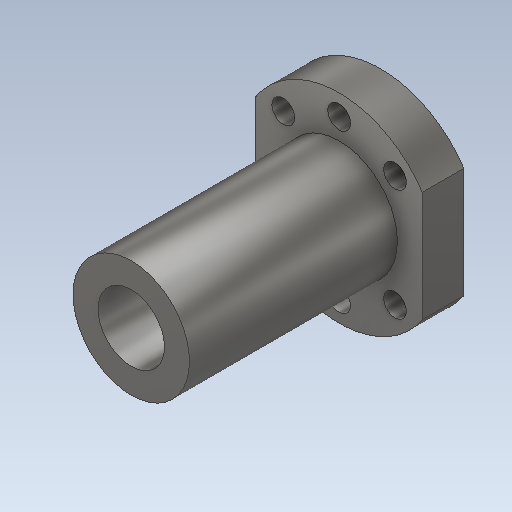
# Autodesk Inventor part: Cartesian1_BallNut
Saved by Autodesk Inventor 2020 (Build 240168000, 168)
## iProperties
Created: 2020-02-29
Part Number: Cartesian1_BallNut
Material: Stal, stopowa
Document SubType Name: Modeling
Designer: invin
Density: 7.73 g/cm^3
Appearance: Częściowo polerowana
Mass: 262.46 g
Surface Area: 125.71 cm^2
Volume: 33.9535 cm^3
Author: invin
Autodesk Inventor part; units mm, degrees
ref_plane "YZ Plane" through (0, 0, 0) normal (1, 0, 0) x (0, 1, 0)
ref_plane "XZ Plane" through (0, 0, 0) normal (0, 1, 0) x (-1, 0, 0)
ref_plane "XY Plane" through (0, 0, 0) normal (0, 0, 1) x (1, 0, 0)
sketch "Szkic1" plane through (0, 0, 0) normal (0, 0, 1) x (1, 0, 0)
  circle A0 centre (0, 0) radius 24
  dimension "d0" = 48
  constraints: 1 centre point, 1 coincident
  measures "d0" diameter of A0
extrude "Wyciągnięcie proste1" add sketch "Szkic1" along normal blind 10
sketch "Szkic2" plane through (0, 0, 10) normal (0, 0, 1) x (1, 0, 0)
  circle A0 centre (0, 0) radius 14
  dimension "d3" = 28
  constraints: 1 centre point, 1 coincident
  measures "d3" diameter of A0
extrude "Wyciągnięcie proste2" add sketch "Szkic2" along normal blind 50
sketch "Szkic3" plane through (0, 0, 60) normal (0, 0, 1) x (1, 0, 0)
  circle A0 centre (0, 0) radius 8
  dimension "d6" = 16
  constraints: 1 centre point, 1 coincident
  measures "d6" diameter of A0
extrude "Wyciągnięcie proste3" cut sketch "Szkic3" against normal through all
sketch "Szkic4" plane through (0, 0, 10) normal (0, 0, 1) x (1, 0, 0)
  line L0 (-34.1509, 26.2264) -> (-20, 26.2264)
  line L1 (-20, 26.2264) -> (-20, -20.7547)
  line L2 (-20, -20.7547) -> (-34.1509, -20.7547)
  line L3 (-34.1509, -20.7547) -> (-34.1509, 26.2264)
  line L4 (20, 30.566) -> (32.0755, 30.566)
  line L5 (32.0755, 30.566) -> (32.0755, -32.8302)
  line L6 (32.0755, -32.8302) -> (20, -32.8302)
  line L7 (20, -32.8302) -> (20, 30.566)
  point P0 (0, 0)
  dimension "d9" = 40
  dimension "d10" = 20
  constraints: 16 end point, 4 parallel, 2 horizontal, 2 perpendicular
  measures "d9" distance between parallel lines of L1 L7
  measures "d10" distance from line of L7 point (0, 0)
extrude "Wyciągnięcie proste4" cut sketch "Szkic4" against normal blind 40
sketch "Szkic5" plane through (0, 0, 10) normal (0, 0, 1) x (1, 0, 0)
  circle A0 centre (0, 0) radius 19
  circle A1 centre (0, 19) radius 2.75
  circle A2 centre (13.435, 13.435) radius 2.75
  circle A3 centre (-13.435, 13.435) radius 2.75
  line L0 (0, 0) -> (-30.3885, 30.3885)
  line L1 (0, 0) -> (37.6377, 37.6377)
  line L2 (0, 0) -> (34.9843, 0)
  dimension "d13" = 38
  dimension "d14" = 5.5
  dimension "d15" = 5.5
  dimension "d16" = 5.5
  dimension "d17" = 45
  dimension "d18" = 90
  constraints: 6 end point, 4 centre point, 3 point on circle, 2 point on line, 1 coincident, 1 horizontal
  measures "d13" diameter of A0
  measures "d14" diameter of A1
  measures "d15" diameter of A2
  measures "d16" diameter of A3
  measures "d17" angle of L2 L1
  measures "d18" angle of L1 L0
extrude "Wyciągnięcie proste5" cut sketch "Szkic5" against normal blind 40 contours A2 L1 A0 | A0 L1 A2 | A3 L0 A0 | A0 L0 A3 | L1 A2 A0 | A0 A2 L1 | L0 A3 A0 | A0 A3 L0 | A1 A0 | A0 A1
mirror "Odbij1" about plane through (0, 0, 0) normal (0, 1, 0) of "Wyciągnięcie proste5"
